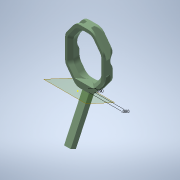
# Autodesk Inventor part: diamond_big_MK
Saved by Autodesk Inventor 2021 (Build 250183000, 183)
## iProperties
Created: 2008-12-01
Part Number: diamond_big_MK
Document SubType Name: Modeling
Designer: osbornej
Density: 1.2 g/cm^3
Material: Polycarbonate, Clear
Mass: 0.27115 g
Surface Area: 4.58727 cm^2
Volume: 0.225958 cm^3
Description: Dudman post #2
Appearance: Green Pastel
Author: osbornej
Autodesk Inventor part; units mm, degrees
sketch "Sketch1" plane through (0, 0, 0) normal (0, 0, 1) x (1, 0, 0)
  line L0 (-2.8702, 9.525) -> (2.8702, 9.525)
  line L1 (6.6802, 4.445) -> (6.6802, -4.445)
  line L2 (2.8702, -9.525) -> (-2.8702, -9.525)
  line L3 (-6.6802, -4.445) -> (-6.6802, 4.445)
  line L4 (-6.6802, -4.445) -> (-2.8702, -9.525)
  line L5 (2.8702, 9.525) -> (6.6802, 4.445)
  line L6 (6.6802, -4.445) -> (2.8702, -9.525)
  line L7 (0, 13.335) -> (0, -13.335) construction
  line L8 (-9.3523, 0) -> (9.3523, 0) construction
  line L9 (-2.8702, 9.525) -> (-6.6802, 4.445)
  line L10 (-4.8765, -3.6735) -> (-4.8765, 3.6735)
  line L11 (-4.8765, 3.6735) -> (-2.0952, 7.3819)
  line L12 (-2.0952, 7.3819) -> (2.0952, 7.3819)
  line L13 (2.0952, 7.3819) -> (4.8765, 3.6735)
  line L14 (4.8765, 3.6735) -> (4.8765, -3.6735)
  line L15 (4.8765, -3.6735) -> (2.0952, -7.3819)
  line L16 (2.0952, -7.3819) -> (-2.0952, -7.3819)
  line L17 (-2.0952, -7.3819) -> (-4.8765, -3.6735)
  dimension "width" = 13.3604
  dimension "d30" = 5.08
  dimension "d41" = 6.6802
  dimension "d72" = 3.81
  dimension "d213" = 19.05
  dimension "d215" = 9.7531
  dimension "d228" = 4.8765
  dimension "d236" = 2.0953
  dimension "d239" = 4.1905
  dimension "d278" = 14.7637
  dimension "d279" = 2.1431
  constraints: 32 end point, 8 parallel, 4 perpendicular, 1 horizontal, 1 vertical, 6 other
  measures "width" distance of L1.end L3.start
  measures "d30" vertical distance of L1.start L0.end
  measures "d41" distance between parallel lines of L7 L3
  measures "d72" distance from line of L0.start L3
  measures "d213" distance between parallel lines of L2 L0
  measures "d215" distance between parallel lines of L14 L10
  measures "d228" distance between parallel lines of L10 L7
  measures "d236" distance from line of L16.end L7
  measures "d239" distance of L11.end L12.end
  measures "d278" distance between parallel lines of L16 L12
  measures "d279" distance between parallel lines of L12 L0
extrude "Extrusion1" add sketch "Sketch1" along normal mid plane 3.175 contours L0 L5 L1 L6 L2 L4 L3 L9 | L10 L11 L12 L13 L14 L15 L16 L17
ref_plane "Work Plane1" through (2.8702, -9.525, 0) normal (0.6, 0.8, 0) x (0, 0, 1)
sketch "Sketch2" plane through (2.8702, -9.525, 0) normal (0.6, 0.8, 0) x (0, 0, 1)
  line L0 (-1.5875, -11.938) -> (-1.5875, 0) projected
  line L1 (-1.5875, 0) -> (1.5875, 0) projected
  line L2 (1.5875, 0) -> (1.5875, -11.938) projected
  line L3 (-1.0817, 0) -> (-0.5556, -1.27)
  line L4 (-0.5556, -1.27) -> (0.5556, -1.27)
  line L5 (-1.5875, -11.938) -> (-1.5875, 0) projected
  line L6 (-1.5875, 0) -> (1.5875, 0) projected
  line L7 (1.5875, 0) -> (1.5875, -11.938) projected
  line L8 (-1.5875, -7.2571) -> (-1.5875, 0)
  line L9 (-1.5875, 0) -> (1.5875, 0)
  line L10 (1.5875, 0) -> (1.5875, -7.2571)
  line L11 (-1.5875, -4.5923) -> (-1.5875, 0) projected
  line L12 (-1.5875, -4.5923) -> (1.5875, -4.5923) projected
  line L13 (1.5875, 0) -> (1.5875, -4.5923) projected
  line L14 (-1.5875, -4.5923) -> (1.5875, -4.5923) projected
  line L15 (-1.5875, -4.5923) -> (-1.5875, 0) projected
  line L16 (-1.5875, 0) -> (1.5875, 0) projected
  line L17 (1.5875, 0) -> (1.5875, -4.5923) projected
  line L18 (1.5875, -7.2571) -> (-1.5875, -7.2571)
  line L19 (0, 7.4717) -> (0, -23.494) projected
  line L20 (0.5556, -1.27) -> (1.0817, 0)
  line L21 (1.0817, 0) -> (-1.0817, 0)
  line L22 (1.5875, -11.938) -> (-1.5875, -11.938) projected
  line L23 (1.5875, -11.938) -> (-1.5875, -11.938) projected
  dimension "d43" = 1.27
  dimension "d46" = 1.1113
  dimension "d47" = 0.5556
  dimension "d48" = 45
  dimension "d49" = 22.5
  constraints: 16 end point, 3 point on line, 1 perpendicular
  measures "d43" distance between parallel lines of L4 L1
  measures "d46" distance of L3.end L4.end
  measures "d47" distance from line of L19 L4.end
  measures "d48" angle of L3 L20
  measures "d49" angle of L3 L19
extrude "Extrusion2" cut sketch "Sketch2" along normal through all both and the other way through all contours L1 L19 L4 L3 | L19 L1 L20 L4
mirror "Mirror3" about plane through (0, 0, 0) normal (0, 1, 0) of "Extrusion2"
mirror "Mirror4" about plane through (0, 0, 0) normal (1, 0, 0) of "Extrusion2", "Mirror3"
ref_plane "Work Plane4" through (2.8702, 9.525, 1.5875) normal (0, 0.2079117, 0.9781476) x (1, 0, 0)
fillet "Fillet1" radius 2.794 16 edges at (-2.8702, 9.525, 1.3346) (-2.8702, 9.525, -1.3346) (2.8702, 9.525, -1.3346) (2.8702, 9.525, 1.3346) (6.6802, 4.445, 1.3346) (6.6802, 4.445, -1.3346) (6.6802, -4.445, -1.3346) (6.6802, -4.445, 1.3346) (2.8702, -9.525, 1.3346) (2.8702, -9.525, -1.3346) (-2.8702, -9.525, -1.3346) (-2.8702, -9.525, 1.3346) (-6.6802, -4.445, 1.3346) (-6.6802, 4.445, 1.3346) (-6.6802, 4.445, -1.3346) (-6.6802, -4.445, -1.3346)
extrude "Extrusion12" cut sketch "Sketch1" along normal through all both and the other way through all contours L10 L11 L12 L13 L14 L15 L16 L17
chamfer "Chamfer5" distance 1.016 angle 45 7 edges at (0, 7.3819, 1.5875) (3.4859, 5.5277, 1.5875) (4.8765, 0, 1.5875) (3.4859, -5.5277, 1.5875) (-4.8765, 0, 1.5875) (-3.4859, 5.5277, 1.5875) (-3.4859, -5.5277, 1.5875)
fillet "Fillet3" radius 3.175 8 edges at (-2.0952, 7.3819, -0.508) (-2.0952, -7.3819, -0.508) (2.0952, -7.3819, -0.508) (4.8765, -3.6735, -0.508) (4.8765, 3.6735, -0.508) (-4.8765, -3.6735, -0.508) (-4.8765, 3.6735, -0.508) (2.0952, 7.3819, -0.508)
fillet "Fillet3" radius 3.175 6 edges at (-2.3492, 7.8899, 1.0795) (-5.3845, 3.8428, 1.0795) (-5.3845, -3.8428, 1.0795) (5.3845, -3.8428, 1.0795) (5.3845, 3.8428, 1.0795) (2.3492, 7.8899, 1.0795)
ref_plane "Work Plane5" through (-2.8702, -9.525, -1.5875) normal (0, -0.8288487, 0.5594729) x (1, 0, 0)
sketch "Sketch24" plane through (6.6802, -2.3283, 0.5556) normal (1, 0, 0) x (0, 0, -1)
  line L0 (0, 11.8533) -> (1.1112, 11.8533) projected
  ellipse E0 centre (2.1431, 3.9031) end of major axis (2.1431, 5.5033) minor radius 0.8128
  line L1 (2.1431, -1.1853) -> (2.1431, 5.842) projected
  dimension "d281" = 1.6002
  dimension "d282" = 0.8128
  dimension "d283" = 7.9502
  constraints: 1 point on line, 2 other
  measures "d283" distance from line of L0 point (2.143, 3.903)
extrude "Extrusion17" cut sketch "Sketch24" against normal blind 25.4
fillet "Fillet8" radius 3.175 4 edges at (5.7784, -0.0254, -1.5875) (5.7535, 3.175, -1.5875) (-5.7535, 3.175, -1.5875) (-5.7784, -0.0254, -1.5875)
ref_plane "Work Plane6" through (-2.8702, -9.525, 1.5875) normal (0, -0.9063078, 0.4226183) x (-1, 0, 0)
sketch "Sketch29" plane through (-2.8702, -9.525, 1.5875) normal (0, -0.9063078, 0.4226183) x (-1, 0, 0)
  line L0 (-3.9938, 0.6012) -> (-1.7078, 0.6012)
  line L1 (-1.7078, 0.6012) -> (-1.7078, 2.6332)
  line L2 (-1.7078, 2.6332) -> (-3.9938, 2.6332)
  line L3 (-3.9938, 2.6332) -> (-3.9938, 0.6012)
  point P0 (-2.8702, -2.5867)
  dimension "d293" = 2.032
  dimension "d294" = 2.286
  constraints: 8 end point, 2 parallel, 1 horizontal, 1 perpendicular
  measures "d293" distance of L2.end L0.start
  measures "d294" distance of L1.end L2.end
extrude "Extrusion20" add sketch "Sketch29" along normal blind 15.24
extrude "Extrusion21" add sketch "Sketch29" against normal blind 1.27
equation "\"d41\" = 0.5 * width"
equation "\"d47\" = 0.5 * d46"
equation "\"d49\" = 0.5 * d48"
equation "\"scale\" = 0.73"
body "Solid1"
